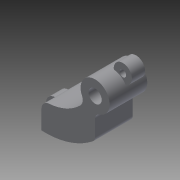
# Autodesk Inventor part: BrakePad
Saved by Autodesk Inventor 2015 (Build 190159000, 159)
## iProperties
Created: 2016-02-14
Part Number: BrakePad
Material: Generic
Document SubType Name: Modeling
Designer: Owner
Density: 1 g/cm^3
Appearance: Default
Author: Owner
Autodesk Inventor part; units mm, degrees
ref_plane "YZ Plane" through (0, 0, 0) normal (1, 0, 0) x (0, 1, 0)
ref_plane "XZ Plane" through (0, 0, 0) normal (0, 1, 0) x (-1, 0, 0)
sketch "Sketch1" plane through (0, 0, 0) normal (0, 0, 1) x (1, 0, 0)
  arc A0 (-0.635, -11.743) -> (7.62, -8.9576) centre (0, 0) ccw
  arc A1 (-0.635, -7.5935) -> (6.0473, -4.6363) centre (0, 0) ccw
  circle A2 centre (7.62, -3.048) radius 2.2352
  line L0 (7.62, -5.2832) -> (7.62, -8.9576)
  line L1 (-0.635, -11.743) -> (-0.635, -7.5935)
  dimension "d3" = 2.2352
  constraints: 6 point on circle, 4 end point, 3 centre point, 1 coincident, 1 parallel, 1 vertical, 1 vertical alignment
  measures "d3" radius of A2
extrude "Extrusion1" add sketch "Sketch1" along normal blind 5.7912
fillet "Fillet2" radius 0.889 2 edges at (7.62, -5.2832, 2.8956) (7.62, -8.9576, 2.8956)
fillet "Fillet3" radius 1.27 2 edges at (6.0473, -4.6363, 2.8956) (-0.635, -7.5935, 2.8956)
ref_plane "Work Plane1" through (0, 0, 1.016) normal (0, 0, -1) x (-1, 0, 0)
sketch "Sketch2" plane through (0, 0, 1.016) normal (0, 0, -1) x (-1, 0, 0)
  line L0 (0, 0) -> (1.27, 0)
  line L1 (1.27, 0) -> (1.27, -10.414)
  circle A0 centre (1.27, -10.414) radius 1.397
  line L2 (0, 0) -> (-9.144, 0)
  line L3 (-9.144, 0) -> (-9.144, -0.635)
  circle A1 centre (-9.144, -0.635) radius 1.397
  dimension "d10" = 1.27
  dimension "d11" = 10.414
  dimension "d12" = 2.794
  dimension "d15" = 9.144
  dimension "d16" = 0.635
  dimension "d17" = 2.794
  constraints: 8 end point, 2 centre point, 2 coincident, 2 horizontal, 2 vertical
  measures "d10" distance of L0.start L0.end
  measures "d11" distance of L0.end L1.end
  measures "d12" diameter of A0
  measures "d15" distance of L0.start L2.end
  measures "d16" distance of L2.end L3.end
  measures "d17" diameter of A1
extrude "Extrusion2" add sketch "Sketch2" against normal blind 2.032
hole "Hole1" at (-1.27, -10.414, 3.048) direction (0, 0, -1) diameter 1.016 end through all
hole "Hole2" at (9.144, -0.635, 3.048) direction (0, 0, -1) diameter 1.016 end through all
hole "Hole3" at (7.62, -3.048, 5.7912) direction (0, 0, -1) diameter 2.032 end through all
body "Solid1"
